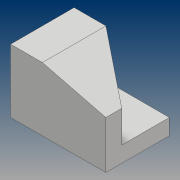
# Autodesk Inventor part: 50 (74000.000 mm^3)
Saved by Autodesk Inventor 2018 (Build 220112000, 112)
## iProperties
Created: 2020-09-18
Part Number: 50 (74000.000 mm^3)
Material: 一般
Document SubType Name: Modeling
Designer: 88697
Density: 1 g/cm^3
Appearance: 預設
Author: 88697
Autodesk Inventor part; units mm, degrees
ref_plane "YZ Plane" through (0, 0, 0) normal (1, 0, 0) x (0, 1, 0)
ref_plane "XZ Plane" through (0, 0, 0) normal (0, 1, 0) x (-1, 0, 0)
sketch "草圖1" plane through (0, 0, 0) normal (0, 1, 0) x (-1, 0, 0)
  line L0 (0, 0) -> (-60, 0)
  line L1 (-60, 0) -> (-60, -40)
  line L2 (-60, -40) -> (0, -40)
  line L3 (0, -40) -> (0, 0)
  dimension "d0" = 60
  dimension "d1" = 40
  constraints: 8 end point, 2 parallel, 1 horizontal, 1 perpendicular
  measures "d0" distance of L0.start L0.end
  measures "d1" distance of L2.end L0.start
extrude "擠出1" add sketch "草圖1" along normal blind 40
sketch "草圖2" plane through (0, 40, 0) normal (0, 1, 0) x (1, 0, 0)
  line L0 (60, 0) -> (60, 40) projected
  line L1 (60, 0) -> (60, 10)
  line L2 (0, 0) -> (60, 0) projected
  line L3 (20, 0) -> (60, 0)
  line L4 (20, 0) -> (60, 10)
  dimension "d5" = 20
  constraints: 6 end point, 1 collinear, 1 horizontal, 1 point on line
  measures "d5" distance of L2.start L3.start
extrude "擠出2" cut sketch "草圖2" against normal blind 40
sketch "草圖3" plane through (0, 40, 0) normal (0, 1, 0) x (1, 0, 0)
  line L0 (60, 40) -> (0, 40) projected
  line L1 (0, 40) -> (0, 0) projected
  line L2 (0, 0) -> (20, 0) projected
  point P0 (20, 30)
  dimension "d8" = 10
  dimension "d9" = 20
  dimension "d10" = 20
  dimension "d11" = 0
  measures "d8" distance from line of L0 point (20, 30)
  measures "d9" distance from line of L1 point (20, 30)
  measures "d10" distance from line of L1 point (20, 0)
  measures "d11" distance from line of L2 point (20, 0)
sketch "草圖4" plane through (60, 0, -40) normal (1, 0, 0) x (0, 0, -1)
  line L0 (-30, 40) -> (-30, 0) projected
  line L1 (-30, 0) -> (0, 0) projected
  point P0 (-40, 0)
  point P1 (-30, 10)
  dimension "d12" = 10
  constraints: 1 point on line
  measures "d12" distance from line of L1 point (-30, 10)
ref_plane "工作平面1" through (20, 40, 0) normal (-0.6, -0.8, 0) x (0, 0, -1)
sketch "草圖5" plane through (20, 40, 0) normal (-0.6, -0.8, 0) x (0, 0, -1)
  line L0 (-51.3035, -32.4862) -> (51.6467, -32.4862)
  line L1 (51.6467, -32.4862) -> (51.6467, 68.0272)
  line L2 (51.6467, 68.0272) -> (-51.3035, 68.0272)
  line L3 (-51.3035, 68.0272) -> (-51.3035, -32.4862)
  point P0 (0, 8)
  constraints: 8 end point, 2 parallel, 1 horizontal, 1 perpendicular
extrude "擠出3" cut sketch "草圖5" against normal blind 40
sketch "草圖6" plane through (60, 0, -10) normal (1, 0, 0) x (0, 0, -1)
  line L0 (30, 0) -> (30, 40) projected
  line L1 (0, 0) -> (30, 0)
  line L2 (30, 0) -> (30, 10)
  line L3 (30, 10) -> (0, 10)
  line L4 (0, 10) -> (0, 0)
  line L5 (30, 0) -> (20, 0)
  line L6 (20, 0) -> (20, 40)
  line L7 (20, 40) -> (30, 40)
  line L8 (30, 40) -> (30, 0)
  line L9 (0, 0) -> (30, 0) projected
  line L10 (-10, 0) -> (-10, 40) projected
  dimension "d15" = 10
  dimension "d16" = 10
  dimension "d17" = 0
  dimension "d18" = 10
  constraints: 16 end point, 4 parallel, 2 horizontal, 2 perpendicular, 1 point on line
  measures "d15" distance between parallel lines of L6 L0
  measures "d16" distance between parallel lines of L1 L3
  measures "d17" distance between parallel lines of L1 L9
  measures "d18" distance between parallel lines of L10 L4
extrude "擠出4" add sketch "草圖6" against normal up to next
